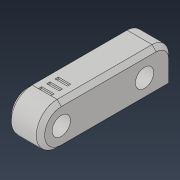
# Autodesk Inventor part: Chipanschlag T1.5
Saved by Autodesk Inventor 2022.2 (Build 262287010, 287A)
## iProperties
Part Number: Chipanschlag T1.5
Material: Generisch
Document SubType Name: Modeling
Designer: rYan
Density: 1 g/cm^3
Appearance: Vorgabe
Author: rYan
Autodesk Inventor part; units mm, degrees
ref_plane "YZ Plane" through (0, 0, 0) normal (1, 0, 0) x (0, 1, 0)
ref_plane "XZ Plane" through (0, 0, 0) normal (0, 1, 0) x (-1, 0, 0)
ref_plane "XY Plane" through (0, 0, 0) normal (0, 0, 1) x (1, 0, 0)
sketch "Skizze1" plane through (0, 0, 0) normal (1, 0, 0) x (0, 1, 0)
  line L0 (0, 0) -> (-10, 0) construction
  circle A0 centre (0, 0) radius 1.1
  circle A1 centre (-10, 0) radius 1.1
  arc A2 (-10, 2.5) -> (-10, -2.5) centre (-10, 0) ccw
  line L1 (-10, -2.5) -> (3.4, -2.5)
  line L2 (-10, 2.5) -> (1.4, 2.5)
  arc A3 (3.4, 0.5) -> (1.4, 2.5) centre (1.4, 0.5) ccw
  line L3 (3.4, 0.5) -> (3.4, -2.5)
  dimension "d0" = 10
  dimension "d1" = 2.2
  dimension "d2" = 2.2
  dimension "d3" = 2.5
  dimension "d8" = 2
  dimension "d9" = 3.4
  constraints: 8 end point, 4 centre point, 4 coincident, 4 point on circle, 4 tangent, 3 horizontal, 1 vertical
  measures "d0" distance of L0.start L0.end
  measures "d1" diameter of A0
  measures "d2" diameter of A1
  measures "d3" radius of A2
  measures "d8" radius of A3
  measures "d9" distance from line of L3 point (0, 0)
extrude "Extrusion1" add sketch "Skizze1" along normal mid plane 4
chamfer "Fase1" distance 0.5 angle 45 10 edges at (2, 2.8142, 1.9142) (2, -4.3, 2.5) (2, -12.5, 0) (2, -3.3, -2.5) (2, 3.4, -1) (-2, 2.8142, 1.9142) (-2, -4.3, 2.5) (-2, -12.5, 0) (-2, -3.3, -2.5) (-2, 3.4, -1)
sketch "Skizze4" plane through (-1.5, -10, 2.5) normal (0, 0, 1) x (1, 0, 0)
  line L0 (1.5, 16.58) -> (1.5, -5.68) construction
  line L1 (0, 0) -> (3, 0) construction
  line L2 (0.75, 0.4) -> (2.25, 0.4)
  line L3 (2.25, 0.4) -> (2.25, 0)
  line L4 (2.25, 0) -> (0.75, 0)
  line L5 (0.75, 0) -> (0.75, 0.4)
  line L6 (0.75, 0.4) -> (2.25, 0) construction
  line L7 (2.25, 0.4) -> (0.75, 0) construction
  point P0 (1.5, 10)
  point P1 (1.5, 0.2)
  point P2 (1.5, 0)
  dimension "d23" = 0.4
  dimension "d24" = 1.5
  constraints: 12 end point, 4 midpoint, 2 parallel, 1 horizontal, 1 perpendicular, 1 point on line
  measures "d23" distance of L2.end L3.end
  measures "d24" distance of L3.end L4.end
extrude "Extrusion3" cut sketch "Skizze4" against normal blind 0.2
pattern_linear "Rechteckige Anordnung1" count 3 spacing 1 along (0, 1, 0) of "Extrusion3"
equation "\"d2\" = d1"
